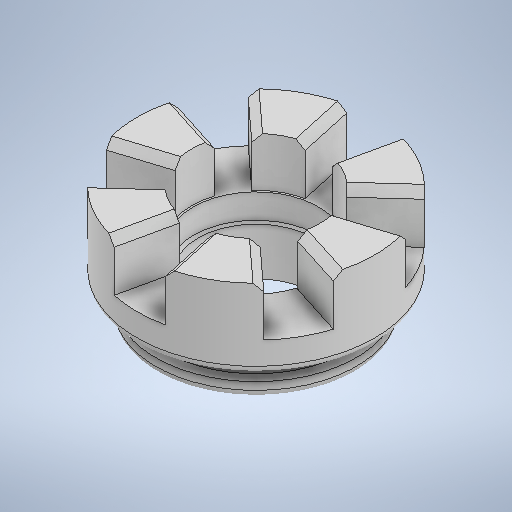
# Autodesk Inventor part: shaft_fixture
Saved by Autodesk Inventor 2025.2 (Build 292293000, 293)
## iProperties
Created: 2025-06-11
Part Number: shaft_fixture
Material: Generic
Document SubType Name: Modeling
Designer: Kacper
Density: 1 g/cm^3
Appearance: Default
Author: Kacper
Autodesk Inventor part; units mm, degrees
ref_plane "YZ Plane" through (0, 0, 0) normal (1, 0, 0) x (0, 1, 0)
ref_plane "XZ Plane" through (0, 0, 0) normal (0, 1, 0) x (-1, 0, 0)
ref_plane "XY Plane" through (0, 0, 0) normal (0, 0, 1) x (1, 0, 0)
sketch "Sketch1" plane through (0, 0, 0) normal (0, 0, 1) x (1, 0, 0)
  line L0 (-31.4382, 0) -> (-31.4382, -8)
  line L1 (-26.5, -13) -> (-26.5, -17)
  line L2 (-26.5, -17) -> (-20.25, -17)
  line L3 (-20.25, -17) -> (-20.25, -19)
  line L4 (-20.25, -19) -> (-15.25, -19)
  line L5 (-15.25, -19) -> (-15.25, -6.5)
  line L6 (-15.25, -6.5) -> (-16.5, -6.5)
  line L7 (-16.5, -6.5) -> (-16.5, 0)
  line L8 (-26.5, -13) -> (-23.9382, -13)
  line L9 (-31.4382, 0) -> (-16.5, 0)
  line L10 (-37.7259, 0) -> (6.2876, 0) projected
  line L11 (-31.4382, -8) -> (-23.9382, -8)
  line L12 (-23.9382, -8) -> (-23.9382, -13)
  line L13 (0, -22.8) -> (0, 3.8) projected
  point P0 (0, 0)
  dimension "d1" = 15.25
  dimension "d2" = 5
  dimension "d3" = 6.25
  dimension "d4" = 2
  dimension "d6" = 4
  dimension "d8" = 8
  dimension "d10" = 6.5
  dimension "d11" = 16.5
  dimension "d12" = 14.9382
  dimension "d14" = 5
  dimension "d15" = 7.5
  constraints: 24 end point, 8 perpendicular, 3 horizontal, 1 collinear, 1 parallel
  measures "d1" horizontal distance of L4.end point (0, 0)
  measures "d2" distance of L3.end L4.end
  measures "d3" distance of L1.end L2.end
  measures "d4" distance of L2.end L3.end
  measures "d6" distance of L1.start L1.end
  measures "d8" distance of L0.start L0.end
  measures "d10" distance of L6.end L7.end
  measures "d11" distance from line of point (0, 0) L7
  measures "d12" distance of L7.end L0.start
  measures "d14" distance of L11.end L8.end
  measures "d15" distance of L0.end L11.end
revolve "Revolution1" add sketch "Sketch1" angle 360 about axis through (0, -10, 0) along (0, 1, 0)
sketch "Sketch2" plane through (0, 0, 0) normal (0, 1, 0) x (1, 0, 0)
  circle A0 centre (0, 0) radius 17 construction
  line L0 (0, 0) -> (-36.8022, 11.7026)
  line L1 (-36.8022, -11.7026) -> (0, 0)
  line L2 (-50.4503, 0) -> (45.0863, 0) projected
  arc A1 (-16.2006, 5.1516) -> (-16.2006, -5.1516) centre (0, 0) ccw
  circle A2 centre (0, 0) radius 31.4382 projected
  arc A3 (-29.96, 9.5269) -> (-29.96, -9.5269) centre (0, 0) ccw
  line L3 (-29.96, -9.5269) -> (-16.2006, -5.1516)
  line L4 (-29.96, 9.5269) -> (-16.2006, 5.1516)
  dimension "d17" = 34
  dimension "d18" = 35.28
  constraints: 8 end point, 8 point on circle, 4 point on line, 3 centre point, 2 collinear, 2 concentric, 1 coincident, 1 other
  measures "d17" diameter of A0
  measures "d18" angle of L0 L1
extrude "Extrusion1" add sketch "Sketch2" along normal blind 13 contours A1 L2 A2 L0 | L1 A2 L2 A1
chamfer "Chamfer1" distance 2 angle 45 2 edges at (-23.0803, 13, -7.3392) (-23.0803, 13, 7.3392)
pattern_circular "Circular Pattern1" count 6 over 360 about axis through (0, -10, 0) along (0, 1, 0) of "Extrusion1", "Chamfer1"
fillet "Fillet1" radius 2 2 edges at (31.4382, -8, 0) (26.5, -17, 0)
body "Solid1"
